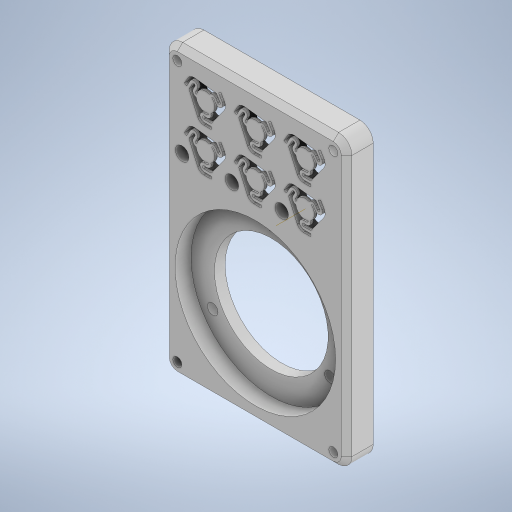
# Autodesk Inventor part: Case Front
Saved by Autodesk Inventor 2023.1 (Build 271208000, 208)
## iProperties
Created: 2022-10-09
Part Number: Case Front
Material: Generic
Document SubType Name: Modeling
Designer: Nick
Density: 1 g/cm^3
Appearance: Default
Author: Nick
Autodesk Inventor part; units mm, degrees
(part 1 of 2)
ref_plane "YZ Plane" through (0, 0, 0) normal (1, 0, 0) x (0, 1, 0)
ref_plane "XZ Plane" through (0, 0, 0) normal (0, 1, 0) x (-1, 0, 0)
ref_plane "XY Plane" through (0, 0, 0) normal (0, 0, 1) x (1, 0, 0)
sketch "Sketch1" plane through (0, 0, 0) normal (0, 0, 1) x (1, 0, 0)
  line L0 (0, 0) -> (68.58, 0)
  line L1 (68.58, 0) -> (68.58, 107.95)
  line L2 (68.58, 107.95) -> (0, 107.95)
  line L3 (0, 107.95) -> (0, 0)
  dimension "d0" = 68.58
  dimension "d1" = 107.95
  constraints: 8 end point, 2 parallel, 1 horizontal, 1 perpendicular
  measures "d0" distance of L2.end L1.end
  measures "d1" distance of L1.end L0.end
extrude "Extrusion1" add sketch "Sketch1" along normal blind 10
sketch "Sketch2" plane through (0, 0, 10) normal (0, 0, 1) x (1, 0, 0)
  circle A0 centre (34.29, 35.56) radius 30.149
  line L0 (0, 0) -> (68.58, 0) projected
  point P0 (34.29, 0)
  dimension "d4" = 60.298
  dimension "d5" = 35.56
  constraints: 1 centre point, 1 midpoint, 1 vertical alignment
  measures "d4" diameter of A0
  measures "d5" distance from line of L0 A0.centre
extrude "Extrusion2" cut sketch "Sketch2" against normal blind 16.9875
sketch "Sketch3" plane through (0, 0, 0) normal (0, 0, -1) x (-1, 0, 0)
  circle A0 centre (-34.29, 35.56) radius 30.149 projected
  circle A1 centre (-34.29, 35.56) radius 21.3606
  point P0 (0, 0)
  dimension "d8" = 42.7212
  constraints: 1 centre point, 1 coincident
  measures "d8" diameter of A1
extrude "Extrusion3" add sketch "Sketch3" against normal blind 4
sketch "Sketch4" plane through (0, 0, 10) normal (0, 0, 1) x (1, 0, 0)
  circle A0 centre (15.59, 78.7495) radius 3
  circle A1 centre (34.29, 78.7495) radius 3
  circle A2 centre (52.99, 94.9095) radius 3
  circle A3 centre (34.29, 94.9095) radius 3
  circle A4 centre (15.59, 94.9095) radius 3
  line L0 (12.59, 97.9095) -> (18.59, 97.9095) construction
  line L1 (18.59, 97.9095) -> (18.59, 91.9095) construction
  line L2 (18.59, 91.9095) -> (12.59, 91.9095) construction
  line L3 (12.59, 91.9095) -> (12.59, 97.9095) construction
  line L4 (31.29, 97.9095) -> (37.29, 97.9095) construction
  line L5 (37.29, 97.9095) -> (37.29, 91.9095) construction
  line L6 (37.29, 91.9095) -> (31.29, 91.9095) construction
  line L7 (31.29, 91.9095) -> (31.29, 97.9095) construction
  line L8 (49.99, 97.9095) -> (55.99, 97.9095) construction
  line L9 (55.99, 97.9095) -> (55.99, 91.9095) construction
  line L10 (55.99, 91.9095) -> (49.99, 91.9095) construction
  line L11 (49.99, 91.9095) -> (49.99, 97.9095) construction
  line L12 (31.29, 81.7495) -> (37.29, 81.7495) construction
  line L13 (37.29, 81.7495) -> (37.29, 75.7495) construction
  line L14 (37.29, 75.7495) -> (31.29, 75.7495) construction
  line L15 (31.29, 75.7495) -> (31.29, 81.7495) construction
  line L16 (12.59, 81.7495) -> (18.59, 81.7495) construction
  line L17 (18.59, 81.7495) -> (18.59, 75.7495) construction
  line L18 (18.59, 75.7495) -> (12.59, 75.7495) construction
  line L19 (12.59, 75.7495) -> (12.59, 81.7495) construction
  line L20 (68.58, 107.95) -> (0, 107.95) construction
  line L21 (17.8543, 65.709) -> (37.2658, 65.709) construction
  circle A5 centre (34.29, 35.56) radius 30.149 construction
  circle A6 centre (52.99, 78.7495) radius 3
  line L22 (49.99, 81.7495) -> (55.99, 81.7495) construction
  line L23 (55.99, 81.7495) -> (55.99, 75.7495) construction
  line L24 (55.99, 75.7495) -> (49.99, 75.7495) construction
  line L25 (49.99, 75.7495) -> (49.99, 81.7495) construction
  line L26 (46.7767, 79.8715) -> (48.1617, 82.2704)
  line L27 (49.2587, 80.1705) -> (49.8937, 81.2704)
  line L28 (45.9106, 80.3715) -> (47.2956, 82.7704)
  line L29 (48.3927, 80.6705) -> (49.0277, 81.7704)
  arc A7 (49.8937, 81.2704) -> (47.2956, 82.7704) centre (48.5947, 82.0204) ccw
  arc A8 (49.0277, 81.7704) -> (48.1617, 82.2704) centre (48.5947, 82.0204) ccw
  arc A9 (48.3927, 80.6705) -> (50.0046, 78.4535) centre (49.6917, 79.9205) ccw
  arc A10 (49.2587, 80.1705) -> (50.1629, 79.7532) centre (49.6917, 79.9205) ccw
  line L30 (52.99, 78.7495) -> (49.5762, 80.7205) construction
  line L31 (52.99, 81.7495) -> (52.99, 78.7495) construction
  line L32 (45.9106, 80.3715) -> (46.7767, 79.8715)
  circle A11 centre (52.99, 78.7495) radius 3.508
  line L33 (46.7767, 79.8715) -> (48.9417, 78.6215)
  line L34 (45.9106, 80.3715) -> (45.0446, 80.8715)
  line L35 (45.0446, 80.8715) -> (46.4296, 83.2704)
  arc A12 (50.7343, 80.7273) -> (46.4296, 83.2704) centre (48.5947, 82.0204) ccw
  point P0 (0, 0)
  point P1 (37.29, 78.7495)
  point P2 (18.59, 78.7495)
  point P3 (18.59, 94.9095)
  point P4 (31.29, 94.9095)
  point P5 (55.99, 94.9095)
  point P6 (34.29, 97.9095)
  point P7 (52.99, 97.9095)
  point P8 (15.59, 97.9095)
  point P9 (15.59, 81.7495)
  point P10 (34.29, 107.95)
  point P11 (55.99, 78.7495)
  point P12 (46.3436, 80.1215)
  point P13 (50.432, 77.1821)
  point P14 (49.5508, 79.4408)
  point P15 (51.0723, 81.6869)
  dimension "d11" = 10.16
  dimension "d12" = 6
  dimension "d13" = 6
  dimension "d14" = 12.7
  dimension "d15" = 12.7
  dimension "d16" = 10.0405
  dimension "d17" = 10.0405
  dimension "d34" = 6
  dimension "d35" = 6
  dimension "d36" = 1
  dimension "d37" = 60
  dimension "d38" = 1.27
  dimension "d58" = 0.508
  dimension "d129" = 1
  dimension "d131" = 1
  constraints: 70 end point, 15 parallel, 15 point on circle, 14 midpoint, 12 centre point, 11 tangent, 10 equal length, 9 perpendicular, 7 horizontal, 7 vertical alignment, 6 horizontal alignment, 5 collinear, 5 equal radius, 3 concentric, 3 point on line, 1 vertical
  measures "d11" distance between parallel lines of L12 L6
  measures "d12" distance of L12.start L12.end
  measures "d13" diameter of A1
  measures "d14" distance between parallel lines of L11 L5
  measures "d15" distance between parallel lines of L1 L7
  measures "d16" distance between parallel lines of L20 L4
  measures "d17" distance between parallel lines of L21 L14
  measures "d34" distance of L25.end L23.start
  measures "d35" diameter of A6
  measures "d36" distance between parallel lines of L27 L29
  measures "d37" angle of L31 L30
  measures "d38" distance of L29.start L29.end
  measures "d58" radial gap between concentric circles of A6 A11
  measures "d129" distance between parallel lines of L29 L26
  measures "d131" distance between parallel lines of L35 L28
extrude "Extrusion5" cut sketch "Sketch4" against normal through all contours A11 A10 L27 A7 L28 L34 L35 A12 | L33 L26 A8 L29 A9
pattern_circular "Circular Pattern2" count 3 over 360 about axis through (52.99, 78.7495, 10) along (0, 0, 1) of "Extrusion5"
sketch "Sketch6" plane through (0, 0, 10) normal (0, 0, 1) x (1, 0, 0)
  line L0 (57.0683, 83.5694) -> (58.4533, 81.1705) projected
  arc A0 (57.5873, 80.6705) -> (58.4533, 81.1705) centre (58.0203, 80.9205) ccw projected
  line L1 (57.5873, 80.6705) -> (56.9523, 81.7704) projected
  arc A1 (56.9523, 81.7704) -> (54.9033, 82.3194) centre (55.6533, 81.0204) ccw projected
  arc A2 (56.0863, 81.2704) -> (55.3083, 81.3823) centre (55.6533, 81.0204) ccw projected
  line L2 (56.0863, 81.2704) -> (56.7213, 80.1705) projected
  arc A3 (56.7213, 80.1705) -> (59.3194, 81.6705) centre (58.0203, 80.9205) ccw projected
  line L3 (59.3194, 81.6705) -> (57.9344, 84.0694) projected
  line L4 (55.125, 72.8076) -> (52.355, 72.8076) projected
  arc A4 (52.355, 73.8076) -> (52.355, 72.8076) centre (52.355, 73.3076) ccw projected
  line L5 (52.355, 73.8076) -> (53.625, 73.8076) projected
  arc A5 (53.625, 73.8076) -> (55.125, 75.3076) centre (53.625, 75.3076) ccw projected
  arc A6 (53.625, 74.8076) -> (54.1109, 75.4254) centre (53.625, 75.3076) ccw projected
  line L6 (53.625, 74.8076) -> (52.355, 74.8076) projected
  arc A7 (52.355, 74.8076) -> (52.355, 71.8076) centre (52.355, 73.3076) ccw projected
  line L7 (52.355, 71.8076) -> (55.125, 71.8076) projected
  line L8 (46.7767, 79.8715) -> (48.1617, 82.2704) projected
  arc A8 (49.0277, 81.7704) -> (48.1617, 82.2704) centre (48.5947, 82.0204) ccw projected
  line L9 (49.0277, 81.7704) -> (48.3927, 80.6705) projected
  arc A9 (48.3927, 80.6705) -> (48.9417, 78.6215) centre (49.6917, 79.9205) ccw projected
  line L10 (47.2956, 82.7704) -> (45.9106, 80.3715) projected
  arc A10 (49.2587, 80.1705) -> (49.5508, 79.4408) centre (49.6917, 79.9205) ccw projected
  line L11 (49.2587, 80.1705) -> (49.8937, 81.2704) projected
  arc A11 (49.8937, 81.2704) -> (47.2956, 82.7704) centre (48.5947, 82.0204) ccw projected
  circle A12 centre (34.29, 35.56) radius 30.149 projected
  line L12 (68.58, 0) -> (68.58, 107.95) projected
  line L13 (68.58, 107.95) -> (0, 107.95) projected
  line L14 (0, 107.95) -> (0, 0) projected
  line L15 (0, 0) -> (68.58, 0) projected
  line L16 (48.8782, 84.5043) -> (57.0683, 83.5694)
  line L17 (46.7767, 79.8715) -> (50.0621, 72.3112)
  line L18 (55.125, 72.8076) -> (60.0297, 79.4331)
  line L19 (54.9033, 82.3194) -> (57.0683, 83.5694) projected
  line L20 (57.9344, 84.0694) -> (58.8004, 84.5694) projected
  line L21 (58.8004, 84.5694) -> (60.1854, 82.1705) projected
  arc A13 (56.4927, 78.9415) -> (60.1854, 82.1705) centre (58.0203, 80.9205) ccw projected
  arc A14 (56.4927, 78.9415) -> (55.3083, 81.3823) centre (52.99, 78.7495) ccw projected
  line L22 (55.125, 75.3076) -> (55.125, 72.8076) projected
  line L23 (55.125, 71.8076) -> (55.125, 70.8076) projected
  line L24 (55.125, 70.8076) -> (52.355, 70.8076) projected
  arc A15 (51.4049, 75.62) -> (52.355, 70.8076) centre (52.355, 73.3076) ccw projected
  arc A16 (51.4049, 75.62) -> (54.1109, 75.4254) centre (52.99, 78.7495) ccw projected
  line L25 (48.9417, 78.6215) -> (46.7767, 79.8715) projected
  line L26 (45.9106, 80.3715) -> (45.0446, 80.8715) projected
  line L27 (45.0446, 80.8715) -> (46.4296, 83.2704) projected
  arc A17 (51.0723, 81.6869) -> (46.4296, 83.2704) centre (48.5947, 82.0204) ccw projected
  arc A18 (51.0723, 81.6869) -> (49.5508, 79.4408) centre (52.99, 78.7495) ccw projected
  arc A19 (51.0723, 81.6869) -> (49.5508, 79.4408) centre (52.99, 78.7495) ccw projected
  arc A20 (51.0723, 81.6869) -> (46.4296, 83.2704) centre (48.5947, 82.0204) ccw projected
  arc A21 (51.4049, 75.62) -> (52.355, 70.8076) centre (52.355, 73.3076) ccw projected
  arc A22 (48.3927, 80.6705) -> (48.9417, 78.6215) centre (49.6917, 79.9205) ccw projected
  arc A23 (48.3927, 80.6705) -> (50.0046, 78.4535) centre (49.6917, 79.9205) ccw projected
  circle A24 centre (52.99, 78.7495) radius 3.508 projected
  point P0 (49.4963, 78.4333)
  constraints: 6 end point, 3 point on circle, 3 tangent, 2 point on line
extrude "Extrusion7" cut sketch "Sketch6" against normal through all contours A24 A15 L17 L25 A23
pattern_circular "Circular Pattern3" count 3 over 360 about axis through (52.99, 78.7495, 10) along (0, 0, 1) of "Extrusion7"
pattern_linear "Rectangular Pattern2" count 3 spacing 18.7 along (-1, 0, 0) count 2 spacing 16.16 along (0, 1, 0) of "Extrusion5", "Circular Pattern2", "Extrusion7", "Circular Pattern3"
sketch "Sketch5" plane through (0, 0, 0) normal (0, 0, -1) x (-1, 0, 0)
  line L0 (-65.58, 104.95) -> (-3, 104.95)
  line L1 (-3, 104.95) -> (-3, 66.587)
  line L2 (-3, 66.587) -> (-65.58, 66.587)
  line L3 (-65.58, 66.587) -> (-65.58, 104.95)
  line L4 (-68.58, 107.95) -> (0, 107.95) projected
  line L5 (0, 107.95) -> (0, 0) projected
  line L6 (-68.58, 0) -> (-68.58, 107.95) projected
  line L7 (-14.955, 70.8076) -> (-17.725, 70.8076) projected
  point P0 (-21.4004, 100.7294)
  point P1 (-21.4004, 100.7294)
  dimension "d52" = 3
  dimension "d53" = 3
  dimension "d54" = 3
  dimension "d74" = 4.2206
  dimension "d136" = 4.2206
  constraints: 8 end point, 2 parallel, 1 coincident, 1 horizontal, 1 perpendicular
  measures "d52" distance between parallel lines of L4 L0
  measures "d53" distance between parallel lines of L5 L1
  measures "d54" distance between parallel lines of L6 L3
  measures "d74" distance from line of L0 point (-21.4, 100.729)
  measures "d136" distance between parallel lines of L2 L7
extrude "Extrusion6" cut sketch "Sketch5" against normal blind 9
sketch "Sketch7" plane through (0, 0, 10) normal (0, 0, 1) x (1, 0, 0)
  line L0 (13.1513, 70.2434) -> (18.0287, 70.2434) construction
  line L1 (18.0287, 70.2434) -> (18.0287, 66.7015) construction
  line L2 (18.0287, 66.7015) -> (13.1513, 66.7015) construction
  line L3 (13.1513, 66.7015) -> (13.1513, 70.2434) construction
  line L4 (31.7583, 70.2434) -> (36.8217, 70.2434) construction
  line L5 (36.8217, 70.2434) -> (36.8217, 66.7015) construction
  line L6 (36.8217, 66.7015) -> (31.7583, 66.7015) construction
  line L7 (31.7583, 66.7015) -> (31.7583, 70.2434) construction
  line L8 (53.7679, 70.2434) -> (52.2121, 70.2434) construction
  line L9 (52.2121, 70.2434) -> (52.2121, 66.7015) construction
  line L10 (52.2121, 66.7015) -> (53.7679, 66.7015) construction
  line L11 (53.7679, 66.7015) -> (53.7679, 70.2434) construction
  line L12 (12.8075, 104.5617) -> (18.3725, 104.5617) construction
  line L13 (18.3725, 104.5617) -> (18.3725, 101.405) construction
  line L14 (18.3725, 101.405) -> (12.8075, 101.405) construction
  line L15 (12.8075, 101.405) -> (12.8075, 104.5617) construction
  line L16 (31.3295, 104.5617) -> (37.2505, 104.5617) construction
  line L17 (37.2505, 104.5617) -> (37.2505, 101.405) construction
  line L18 (37.2505, 101.405) -> (31.3295, 101.405) construction
  line L19 (31.3295, 101.405) -> (31.3295, 104.5617) construction
  line L20 (49.6833, 104.5617) -> (56.2967, 104.5617) construction
  line L21 (56.2967, 104.5617) -> (56.2967, 101.405) construction
  line L22 (56.2967, 101.405) -> (49.6833, 101.405) construction
  line L23 (49.6833, 101.405) -> (49.6833, 104.5617) construction
  line L24 (68.58, 0) -> (68.58, 107.95) projected
  line L25 (68.58, 107.95) -> (0, 107.95) projected
  line L26 (0, 107.95) -> (0, 0) projected
  line L27 (0, 0) -> (68.58, 0) projected
  circle A0 centre (34.29, 35.56) radius 30.149 projected
  line L28 (57.0683, 83.5694) -> (58.4533, 81.1705) projected
  arc A1 (57.5873, 80.6705) -> (58.4533, 81.1705) centre (58.0203, 80.9205) ccw projected
  line L29 (57.5873, 80.6705) -> (56.9523, 81.7704) projected
  arc A2 (56.9523, 81.7704) -> (54.463, 81.9332) centre (55.6533, 81.0204) ccw projected
  arc A3 (49.2587, 80.1705) -> (49.5508, 79.4408) centre (49.6917, 79.9205) ccw projected
  line L30 (49.2587, 80.1705) -> (49.8937, 81.2704) projected
  arc A4 (49.8937, 81.2704) -> (47.2956, 82.7704) centre (48.5947, 82.0204) ccw projected
  line L31 (47.2956, 82.7704) -> (45.9106, 80.3715) projected
  line L32 (55.125, 72.8076) -> (52.355, 72.8076) projected
  arc A5 (52.355, 73.8076) -> (52.355, 72.8076) centre (52.355, 73.3076) ccw projected
  line L33 (52.355, 73.8076) -> (53.625, 73.8076) projected
  arc A6 (53.625, 73.8076) -> (55.0107, 75.8819) centre (53.625, 75.3076) ccw projected
  arc A7 (56.0863, 81.2704) -> (55.3083, 81.3823) centre (55.6533, 81.0204) ccw projected
  line L34 (56.0863, 81.2704) -> (56.7213, 80.1705) projected
  arc A8 (56.7213, 80.1705) -> (59.3194, 81.6705) centre (58.0203, 80.9205) ccw projected
  line L35 (59.3194, 81.6705) -> (57.9344, 84.0694) projected
  line L36 (46.7767, 79.8715) -> (48.1617, 82.2704) projected
  arc A9 (49.0277, 81.7704) -> (48.1617, 82.2704) centre (48.5947, 82.0204) ccw projected
  line L37 (49.0277, 81.7704) -> (48.3927, 80.6705) projected
  arc A10 (48.3927, 80.6705) -> (49.4963, 78.4333) centre (49.6917, 79.9205) ccw projected
  arc A11 (53.625, 74.8076) -> (54.1109, 75.4254) centre (53.625, 75.3076) ccw projected
  line L38 (53.625, 74.8076) -> (52.355, 74.8076) projected
  arc A12 (52.355, 74.8076) -> (52.355, 71.8076) centre (52.355, 73.3076) ccw projected
  line L39 (52.355, 71.8076) -> (55.125, 71.8076) projected
  arc A13 (34.925, 74.8076) -> (35.4109, 75.4254) centre (34.925, 75.3076) ccw projected
  line L40 (34.925, 74.8076) -> (33.655, 74.8076) projected
  arc A14 (33.655, 74.8076) -> (33.655, 71.8076) centre (33.655, 73.3076) ccw projected
  line L41 (33.655, 71.8076) -> (36.425, 71.8076) projected
  line L42 (28.0767, 79.8715) -> (29.4617, 82.2704) projected
  arc A15 (30.3277, 81.7704) -> (29.4617, 82.2704) centre (29.8947, 82.0204) ccw projected
  line L43 (30.3277, 81.7704) -> (29.6927, 80.6705) projected
  arc A16 (29.6927, 80.6705) -> (30.7963, 78.4333) centre (30.9917, 79.9205) ccw projected
  arc A17 (37.3863, 81.2704) -> (36.6083, 81.3823) centre (36.9533, 81.0204) ccw projected
  line L44 (37.3863, 81.2704) -> (38.0213, 80.1705) projected
  arc A18 (38.0213, 80.1705) -> (40.6194, 81.6705) centre (39.3203, 80.9205) ccw projected
  line L45 (40.6194, 81.6705) -> (39.2344, 84.0694) projected
  line L46 (36.425, 72.8076) -> (33.655, 72.8076) projected
  arc A19 (33.655, 73.8076) -> (33.655, 72.8076) centre (33.655, 73.3076) ccw projected
  line L47 (33.655, 73.8076) -> (34.925, 73.8076) projected
  arc A20 (34.925, 73.8076) -> (36.3107, 75.8819) centre (34.925, 75.3076) ccw projected
  line L48 (38.3683, 83.5694) -> (39.7533, 81.1705) projected
  arc A21 (38.8873, 80.6705) -> (39.7533, 81.1705) centre (39.3203, 80.9205) ccw projected
  line L49 (38.8873, 80.6705) -> (38.2523, 81.7704) projected
  arc A22 (38.2523, 81.7704) -> (35.763, 81.9332) centre (36.9533, 81.0204) ccw projected
  arc A23 (30.5587, 80.1705) -> (30.8508, 79.4408) centre (30.9917, 79.9205) ccw projected
  line L50 (30.5587, 80.1705) -> (31.1937, 81.2704) projected
  arc A24 (31.1937, 81.2704) -> (28.5956, 82.7704) centre (29.8947, 82.0204) ccw projected
  line L51 (28.5956, 82.7704) -> (27.2106, 80.3715) projected
  arc A25 (16.225, 74.8076) -> (16.7109, 75.4254) centre (16.225, 75.3076) ccw projected
  line L52 (16.225, 74.8076) -> (14.955, 74.8076) projected
  arc A26 (14.955, 74.8076) -> (14.955, 71.8076) centre (14.955, 73.3076) ccw projected
  line L53 (14.955, 71.8076) -> (17.725, 71.8076) projected
  line L54 (9.3767, 79.8715) -> (10.7617, 82.2704) projected
  arc A27 (11.6277, 81.7704) -> (10.7617, 82.2704) centre (11.1947, 82.0204) ccw projected
  line L55 (11.6277, 81.7704) -> (10.9927, 80.6705) projected
  arc A28 (10.9927, 80.6705) -> (12.0963, 78.4333) centre (12.2917, 79.9205) ccw projected
  arc A29 (18.6863, 81.2704) -> (17.9083, 81.3823) centre (18.2533, 81.0204) ccw projected
  line L56 (18.6863, 81.2704) -> (19.3213, 80.1705) projected
  arc A30 (19.3213, 80.1705) -> (21.9194, 81.6705) centre (20.6203, 80.9205) ccw projected
  line L57 (21.9194, 81.6705) -> (20.5344, 84.0694) projected
  line L58 (17.725, 72.8076) -> (14.955, 72.8076) projected
  arc A31 (14.955, 73.8076) -> (14.955, 72.8076) centre (14.955, 73.3076) ccw projected
  line L59 (14.955, 73.8076) -> (16.225, 73.8076) projected
  arc A32 (16.225, 73.8076) -> (17.6107, 75.8819) centre (16.225, 75.3076) ccw projected
  line L60 (19.6683, 83.5694) -> (21.0533, 81.1705) projected
  arc A33 (20.1873, 80.6705) -> (21.0533, 81.1705) centre (20.6203, 80.9205) ccw projected
  line L61 (20.1873, 80.6705) -> (19.5523, 81.7704) projected
  arc A34 (19.5523, 81.7704) -> (17.063, 81.9332) centre (18.2533, 81.0204) ccw projected
  arc A35 (11.8587, 80.1705) -> (12.1508, 79.4408) centre (12.2917, 79.9205) ccw projected
  line L62 (11.8587, 80.1705) -> (12.4937, 81.2704) projected
  arc A36 (12.4937, 81.2704) -> (9.8956, 82.7704) centre (11.1947, 82.0204) ccw projected
  line L63 (9.8956, 82.7704) -> (8.5106, 80.3715) projected
  arc A37 (53.625, 90.9676) -> (54.1109, 91.5854) centre (53.625, 91.4676) ccw projected
  line L64 (53.625, 90.9676) -> (52.355, 90.9676) projected
  arc A38 (52.355, 90.9676) -> (52.355, 87.9676) centre (52.355, 89.4676) ccw projected
  line L65 (52.355, 87.9676) -> (55.125, 87.9676) projected
  line L66 (46.7767, 96.0315) -> (48.1617, 98.4304) projected
  arc A39 (49.0277, 97.9304) -> (48.1617, 98.4304) centre (48.5947, 98.1804) ccw projected
  line L67 (49.0277, 97.9304) -> (48.3927, 96.8305) projected
  arc A40 (48.3927, 96.8305) -> (49.4963, 94.5933) centre (49.6917, 96.0805) ccw projected
  arc A41 (56.0863, 97.4304) -> (55.3083, 97.5423) centre (55.6533, 97.1804) ccw projected
  line L68 (56.0863, 97.4304) -> (56.7213, 96.3305) projected
  arc A42 (56.7213, 96.3305) -> (59.3194, 97.8305) centre (58.0203, 97.0805) ccw projected
  line L69 (59.3194, 97.8305) -> (57.9344, 100.2294) projected
  line L70 (55.125, 88.9676) -> (52.355, 88.9676) projected
  arc A43 (52.355, 89.9676) -> (52.355, 88.9676) centre (52.355, 89.4676) ccw projected
  line L71 (52.355, 89.9676) -> (53.625, 89.9676) projected
  arc A44 (53.625, 89.9676) -> (55.0107, 92.0419) centre (53.625, 91.4676) ccw projected
  line L72 (57.0683, 99.7294) -> (58.4533, 97.3305) projected
  arc A45 (57.5873, 96.8305) -> (58.4533, 97.3305) centre (58.0203, 97.0805) ccw projected
  line L73 (57.5873, 96.8305) -> (56.9523, 97.9304) projected
  arc A46 (56.9523, 97.9304) -> (54.463, 98.0932) centre (55.6533, 97.1804) ccw projected
  arc A47 (49.2587, 96.3305) -> (49.5508, 95.6008) centre (49.6917, 96.0805) ccw projected
  line L74 (49.2587, 96.3305) -> (49.8937, 97.4304) projected
  arc A48 (49.8937, 97.4304) -> (47.2956, 98.9304) centre (48.5947, 98.1804) ccw projected
  line L75 (47.2956, 98.9304) -> (45.9106, 96.5315) projected
  arc A49 (34.925, 90.9676) -> (35.4109, 91.5854) centre (34.925, 91.4676) ccw projected
  line L76 (34.925, 90.9676) -> (33.655, 90.9676) projected
  arc A50 (33.655, 90.9676) -> (33.655, 87.9676) centre (33.655, 89.4676) ccw projected
  line L77 (33.655, 87.9676) -> (36.425, 87.9676) projected
  line L78 (28.0767, 96.0315) -> (29.4617, 98.4304) projected
  arc A51 (30.3277, 97.9304) -> (29.4617, 98.4304) centre (29.8947, 98.1804) ccw projected
  line L79 (30.3277, 97.9304) -> (29.6927, 96.8305) projected
  arc A52 (29.6927, 96.8305) -> (30.7963, 94.5933) centre (30.9917, 96.0805) ccw projected
  arc A53 (37.3863, 97.4304) -> (36.6083, 97.5423) centre (36.9533, 97.1804) ccw projected
  line L80 (37.3863, 97.4304) -> (38.0213, 96.3305) projected
  arc A54 (38.0213, 96.3305) -> (40.6194, 97.8305) centre (39.3203, 97.0805) ccw projected
  line L81 (40.6194, 97.8305) -> (39.2344, 100.2294) projected
  line L82 (36.425, 88.9676) -> (33.655, 88.9676) projected
  arc A55 (33.655, 89.9676) -> (33.655, 88.9676) centre (33.655, 89.4676) ccw projected
  line L83 (33.655, 89.9676) -> (34.925, 89.9676) projected
  arc A56 (34.925, 89.9676) -> (36.3107, 92.0419) centre (34.925, 91.4676) ccw projected
  line L84 (38.3683, 99.7294) -> (39.7533, 97.3305) projected
  arc A57 (38.8873, 96.8305) -> (39.7533, 97.3305) centre (39.3203, 97.0805) ccw projected
  line L85 (38.8873, 96.8305) -> (38.2523, 97.9304) projected
  arc A58 (38.2523, 97.9304) -> (35.763, 98.0932) centre (36.9533, 97.1804) ccw projected
  arc A59 (30.5587, 96.3305) -> (30.8508, 95.6008) centre (30.9917, 96.0805) ccw projected
  line L86 (30.5587, 96.3305) -> (31.1937, 97.4304) projected
  arc A60 (31.1937, 97.4304) -> (28.5956, 98.9304) centre (29.8947, 98.1804) ccw projected
  line L87 (28.5956, 98.9304) -> (27.2106, 96.5315) projected
  arc A61 (16.225, 90.9676) -> (16.7109, 91.5854) centre (16.225, 91.4676) ccw projected
  line L88 (16.225, 90.9676) -> (14.955, 90.9676) projected
  arc A62 (14.955, 90.9676) -> (14.955, 87.9676) centre (14.955, 89.4676) ccw projected
  line L89 (14.955, 87.9676) -> (17.725, 87.9676) projected
  line L90 (9.3767, 96.0315) -> (10.7617, 98.4304) projected
  arc A63 (11.6277, 97.9304) -> (10.7617, 98.4304) centre (11.1947, 98.1804) ccw projected
  line L91 (11.6277, 97.9304) -> (10.9927, 96.8305) projected
  arc A64 (10.9927, 96.8305) -> (12.0963, 94.5933) centre (12.2917, 96.0805) ccw projected
  arc A65 (18.6863, 97.4304) -> (17.9083, 97.5423) centre (18.2533, 97.1804) ccw projected
  line L92 (18.6863, 97.4304) -> (19.3213, 96.3305) projected
  arc A66 (19.3213, 96.3305) -> (21.9194, 97.8305) centre (20.6203, 97.0805) ccw projected
  line L93 (21.9194, 97.8305) -> (20.5344, 100.2294) projected
  line L94 (17.725, 88.9676) -> (14.955, 88.9676) projected
  arc A67 (14.955, 89.9676) -> (14.955, 88.9676) centre (14.955, 89.4676) ccw projected
  line L95 (14.955, 89.9676) -> (16.225, 89.9676) projected
  arc A68 (16.225, 89.9676) -> (17.6107, 92.0419) centre (16.225, 91.4676) ccw projected
  line L96 (19.6683, 99.7294) -> (21.0533, 97.3305) projected
  arc A69 (20.1873, 96.8305) -> (21.0533, 97.3305) centre (20.6203, 97.0805) ccw projected
  line L97 (20.1873, 96.8305) -> (19.5523, 97.9304) projected
  arc A70 (19.5523, 97.9304) -> (17.063, 98.0932) centre (18.2533, 97.1804) ccw projected
  arc A71 (11.8587, 96.3305) -> (12.1508, 95.6008) centre (12.2917, 96.0805) ccw projected
  line L98 (11.8587, 96.3305) -> (12.4937, 97.4304) projected
  arc A72 (12.4937, 97.4304) -> (9.8956, 98.9304) centre (11.1947, 98.1804) ccw projected
  line L99 (9.8956, 98.9304) -> (8.5106, 96.5315) projected
  circle A73 centre (6.7912, 73.6695) radius 2.55
  circle A74 centre (25.4912, 73.6695) radius 2.55
  circle A75 centre (44.1912, 73.6695) radius 2.55
  line L100 (15.59, 78.7495) -> (52.99, 78.7495) construction
  line L101 (15.59, 78.7495) -> (6.7912, 73.6695) construction
  line L102 (52.99, 78.7495) -> (44.1912, 73.6695) construction
  line L103 (55.125, 71.8076) -> (55.125, 70.8076) projected
  line L104 (55.125, 70.8076) -> (52.355, 70.8076) projected
  arc A76 (50.0621, 72.3112) -> (52.355, 70.8076) centre (52.355, 73.3076) ccw projected
  line L105 (45.9106, 80.3715) -> (45.0446, 80.8715) projected
  line L106 (45.0446, 80.8715) -> (46.4296, 83.2704) projected
  arc A77 (48.8782, 84.5043) -> (46.4296, 83.2704) centre (48.5947, 82.0204) ccw projected
  line L107 (57.9344, 84.0694) -> (58.8004, 84.5694) projected
  line L108 (58.8004, 84.5694) -> (60.1854, 82.1705) projected
  arc A78 (60.0297, 79.4331) -> (60.1854, 82.1705) centre (58.0203, 80.9205) ccw projected
  arc A79 (35.763, 81.9332) -> (30.8508, 79.4408) centre (34.29, 78.7495) ccw projected
  line L109 (36.425, 71.8076) -> (36.425, 70.8076) projected
  line L110 (36.425, 70.8076) -> (33.655, 70.8076) projected
  arc A80 (31.3621, 72.3112) -> (33.655, 70.8076) centre (33.655, 73.3076) ccw projected
  line L111 (27.2106, 80.3715) -> (26.3446, 80.8715) projected
  line L112 (26.3446, 80.8715) -> (27.7296, 83.2704) projected
  arc A81 (30.1782, 84.5043) -> (27.7296, 83.2704) centre (29.8947, 82.0204) ccw projected
  line L113 (39.2344, 84.0694) -> (40.1004, 84.5694) projected
  line L114 (40.1004, 84.5694) -> (41.4854, 82.1705) projected
  arc A82 (41.3297, 79.4331) -> (41.4854, 82.1705) centre (39.3203, 80.9205) ccw projected
  arc A83 (17.063, 81.9332) -> (12.1508, 79.4408) centre (15.59, 78.7495) ccw projected
  line L115 (17.725, 71.8076) -> (17.725, 70.8076) projected
  line L116 (17.725, 70.8076) -> (14.955, 70.8076) projected
  arc A84 (12.6621, 72.3112) -> (14.955, 70.8076) centre (14.955, 73.3076) ccw projected
  line L117 (8.5106, 80.3715) -> (7.6446, 80.8715) projected
  line L118 (7.6446, 80.8715) -> (9.0296, 83.2704) projected
  arc A85 (11.4782, 84.5043) -> (9.0296, 83.2704) centre (11.1947, 82.0204) ccw projected
  line L119 (20.5344, 84.0694) -> (21.4004, 84.5694) projected
  line L120 (21.4004, 84.5694) -> (22.7854, 82.1705) projected
  arc A86 (22.6297, 79.4331) -> (22.7854, 82.1705) centre (20.6203, 80.9205) ccw projected
  arc A87 (54.463, 98.0932) -> (49.5508, 95.6008) centre (52.99, 94.9095) ccw projected
  line L121 (55.125, 87.9676) -> (55.125, 86.9676) projected
  line L122 (55.125, 86.9676) -> (52.355, 86.9676) projected
  arc A88 (50.0621, 88.4712) -> (52.355, 86.9676) centre (52.355, 89.4676) ccw projected
  line L123 (45.9106, 96.5315) -> (45.0446, 97.0315) projected
  line L124 (45.0446, 97.0315) -> (46.4296, 99.4304) projected
  arc A89 (48.8782, 100.6643) -> (46.4296, 99.4304) centre (48.5947, 98.1804) ccw projected
  line L125 (57.9344, 100.2294) -> (58.8004, 100.7294) projected
  line L126 (58.8004, 100.7294) -> (60.1854, 98.3305) projected
  arc A90 (60.0297, 95.5931) -> (60.1854, 98.3305) centre (58.0203, 97.0805) ccw projected
  arc A91 (35.763, 98.0932) -> (30.8508, 95.6008) centre (34.29, 94.9095) ccw projected
  line L127 (36.425, 87.9676) -> (36.425, 86.9676) projected
  line L128 (36.425, 86.9676) -> (33.655, 86.9676) projected
  arc A92 (31.3621, 88.4712) -> (33.655, 86.9676) centre (33.655, 89.4676) ccw projected
  line L129 (27.2106, 96.5315) -> (26.3446, 97.0315) projected
  line L130 (26.3446, 97.0315) -> (27.7296, 99.4304) projected
  arc A93 (30.1782, 100.6643) -> (27.7296, 99.4304) centre (29.8947, 98.1804) ccw projected
  line L131 (39.2344, 100.2294) -> (40.1004, 100.7294) projected
  line L132 (40.1004, 100.7294) -> (41.4854, 98.3305) projected
  arc A94 (41.3297, 95.5931) -> (41.4854, 98.3305) centre (39.3203, 97.0805) ccw projected
  arc A95 (17.063, 98.0932) -> (12.1508, 95.6008) centre (15.59, 94.9095) ccw projected
  line L133 (17.725, 87.9676) -> (17.725, 86.9676) projected
  line L134 (17.725, 86.9676) -> (14.955, 86.9676) projected
  arc A96 (12.6621, 88.4712) -> (14.955, 86.9676) centre (14.955, 89.4676) ccw projected
  line L135 (8.5106, 96.5315) -> (7.6446, 97.0315) projected
  line L136 (7.6446, 97.0315) -> (9.0296, 99.4304) projected
  arc A97 (11.4782, 100.6643) -> (9.0296, 99.4304) centre (11.1947, 98.1804) ccw projected
  line L137 (20.5344, 100.2294) -> (21.4004, 100.7294) projected
  line L138 (21.4004, 100.7294) -> (22.7854, 98.3305) projected
  arc A98 (22.6297, 95.5931) -> (22.7854, 98.3305) centre (20.6203, 97.0805) ccw projected
  arc A99 (12.0963, 94.5933) -> (16.7109, 91.5854) centre (15.59, 94.9095) ccw projected
  line L139 (12.6621, 88.4712) -> (9.3767, 96.0315) projected
  arc A100 (30.7963, 94.5933) -> (35.4109, 91.5854) centre (34.29, 94.9095) ccw projected
  line L140 (31.3621, 88.4712) -> (28.0767, 96.0315) projected
  arc A101 (49.4963, 94.5933) -> (54.1109, 91.5854) centre (52.99, 94.9095) ccw projected
  line L141 (50.0621, 88.4712) -> (46.7767, 96.0315) projected
  arc A102 (12.0963, 78.4333) -> (16.7109, 75.4254) centre (15.59, 78.7495) ccw projected
  line L142 (12.6621, 72.3112) -> (9.3767, 79.8715) projected
  arc A103 (30.7963, 78.4333) -> (35.4109, 75.4254) centre (34.29, 78.7495) ccw projected
  line L143 (31.3621, 72.3112) -> (28.0767, 79.8715) projected
  arc A104 (17.6107, 92.0419) -> (17.9083, 97.5423) centre (15.59, 94.9095) ccw projected
  arc A105 (36.3107, 92.0419) -> (36.6083, 97.5423) centre (34.29, 94.9095) ccw projected
  arc A106 (55.0107, 92.0419) -> (55.3083, 97.5423) centre (52.99, 94.9095) ccw projected
  arc A107 (17.6107, 75.8819) -> (17.9083, 81.3823) centre (15.59, 78.7495) ccw projected
  arc A108 (36.3107, 75.8819) -> (36.6083, 81.3823) centre (34.29, 78.7495) ccw projected
  arc A109 (54.463, 81.9332) -> (49.5508, 79.4408) centre (52.99, 78.7495) ccw projected
  line L144 (48.8782, 84.5043) -> (57.0683, 83.5694) projected
  arc A110 (55.0107, 75.8819) -> (55.3083, 81.3823) centre (52.99, 78.7495) ccw projected
  line L145 (60.0297, 79.4331) -> (55.125, 72.8076) projected
  line L146 (50.0621, 72.3112) -> (46.7767, 79.8715) projected
  arc A111 (49.4963, 78.4333) -> (54.1109, 75.4254) centre (52.99, 78.7495) ccw projected
  line L147 (25.4912, 73.6695) -> (34.29, 78.7495) construction
  line L148 (11.4782, 100.6643) -> (19.6683, 99.7294) projected
  line L149 (22.6297, 95.5931) -> (17.725, 88.9676) projected
  line L150 (30.1782, 100.6643) -> (38.3683, 99.7294) projected
  line L151 (41.3297, 95.5931) -> (36.425, 88.9676) projected
  line L152 (48.8782, 100.6643) -> (57.0683, 99.7294) projected
  line L153 (60.0297, 95.5931) -> (55.125, 88.9676) projected
  line L154 (11.4782, 84.5043) -> (19.6683, 83.5694) projected
  line L155 (22.6297, 79.4331) -> (17.725, 72.8076) projected
  line L156 (30.1782, 84.5043) -> (38.3683, 83.5694) projected
  line L157 (41.3297, 79.4331) -> (36.425, 72.8076) projected
  point P0 (52.99, 101.405)
  point P1 (34.29, 101.405)
  point P2 (15.59, 101.405)
  point P3 (34.29, 70.2434)
  point P4 (52.99, 70.2434)
  point P5 (15.59, 70.2434)
  dimension "d0" = 68.58
  dimension "d1" = 107.95
  dimension "d63" = 5.1
  dimension "d64" = 30
  dimension "d66" = 30
  dimension "d137" = 10.16
  constraints: 8 collinear, 8 end point, 8 vertical alignment, 7 midpoint, 3 centre point, 3 parallel, 2 coincident, 2 equal radius, 1 horizontal, 1 point on line, 12 other
  measures "d63" diameter of A73
  measures "d64" angle of L100 L102
  measures "d66" angle of L100 L101
  measures "d137" distance of L147.start L147.end
extrude "Extrusion8" cut sketch "Sketch7" against normal through all contours A73 | A74 | A75
sketch "Sketch8" plane through (0, 0, 9) normal (0, 0, -1) x (-1, 0, 0)
  circle A0 centre (-6.7912, 73.6695) radius 2.55 projected
  circle A1 centre (-44.1912, 73.6695) radius 2.55 projected
  circle A2 centre (-25.4912, 73.6695) radius 2.55 projected
  line L0 (-14.955, 87.9676) -> (-17.725, 87.9676) projected
  arc A3 (-14.955, 87.9676) -> (-14.955, 90.9676) centre (-14.955, 89.4676) ccw projected
  line L1 (-16.225, 90.9676) -> (-14.955, 90.9676) projected
  arc A4 (-16.7109, 91.5854) -> (-16.225, 90.9676) centre (-16.225, 91.4676) ccw projected
  arc A5 (-12.0963, 94.5933) -> (-10.9927, 96.8305) centre (-12.2917, 96.0805) ccw projected
  line L2 (-11.6277, 97.9304) -> (-10.9927, 96.8305) projected
  arc A6 (-10.7617, 98.4304) -> (-11.6277, 97.9304) centre (-11.1947, 98.1804) ccw projected
  line L3 (-9.3767, 96.0315) -> (-10.7617, 98.4304) projected
  line L4 (-21.9194, 97.8305) -> (-20.5344, 100.2294) projected
  arc A7 (-21.9194, 97.8305) -> (-19.3213, 96.3305) centre (-20.6203, 97.0805) ccw projected
  line L5 (-18.6863, 97.4304) -> (-19.3213, 96.3305) projected
  arc A8 (-17.9083, 97.5423) -> (-18.6863, 97.4304) centre (-18.2533, 97.1804) ccw projected
  arc A9 (-17.6107, 92.0419) -> (-16.225, 89.9676) centre (-16.225, 91.4676) ccw projected
  line L6 (-14.955, 89.9676) -> (-16.225, 89.9676) projected
  arc A10 (-14.955, 88.9676) -> (-14.955, 89.9676) centre (-14.955, 89.4676) ccw projected
  line L7 (-17.725, 88.9676) -> (-14.955, 88.9676) projected
  line L8 (-9.8956, 98.9304) -> (-8.5106, 96.5315) projected
  arc A11 (-9.8956, 98.9304) -> (-12.4937, 97.4304) centre (-11.1947, 98.1804) ccw projected
  line L9 (-11.8587, 96.3305) -> (-12.4937, 97.4304) projected
  arc A12 (-12.1508, 95.6008) -> (-11.8587, 96.3305) centre (-12.2917, 96.0805) ccw projected
  arc A13 (-17.063, 98.0932) -> (-19.5523, 97.9304) centre (-18.2533, 97.1804) ccw projected
  line L10 (-20.1873, 96.8305) -> (-19.5523, 97.9304) projected
  arc A14 (-21.0533, 97.3305) -> (-20.1873, 96.8305) centre (-20.6203, 97.0805) ccw projected
  line L11 (-19.6683, 99.7294) -> (-21.0533, 97.3305) projected
  line L12 (-33.655, 87.9676) -> (-36.425, 87.9676) projected
  arc A15 (-33.655, 87.9676) -> (-33.655, 90.9676) centre (-33.655, 89.4676) ccw projected
  line L13 (-34.925, 90.9676) -> (-33.655, 90.9676) projected
  arc A16 (-35.4109, 91.5854) -> (-34.925, 90.9676) centre (-34.925, 91.4676) ccw projected
  arc A17 (-30.7963, 94.5933) -> (-29.6927, 96.8305) centre (-30.9917, 96.0805) ccw projected
  line L14 (-30.3277, 97.9304) -> (-29.6927, 96.8305) projected
  arc A18 (-29.4617, 98.4304) -> (-30.3277, 97.9304) centre (-29.8947, 98.1804) ccw projected
  line L15 (-28.0767, 96.0315) -> (-29.4617, 98.4304) projected
  line L16 (-40.6194, 97.8305) -> (-39.2344, 100.2294) projected
  arc A19 (-40.6194, 97.8305) -> (-38.0213, 96.3305) centre (-39.3203, 97.0805) ccw projected
  line L17 (-37.3863, 97.4304) -> (-38.0213, 96.3305) projected
  arc A20 (-36.6083, 97.5423) -> (-37.3863, 97.4304) centre (-36.9533, 97.1804) ccw projected
  arc A21 (-36.3107, 92.0419) -> (-34.925, 89.9676) centre (-34.925, 91.4676) ccw projected
  line L18 (-33.655, 89.9676) -> (-34.925, 89.9676) projected
  arc A22 (-33.655, 88.9676) -> (-33.655, 89.9676) centre (-33.655, 89.4676) ccw projected
  line L19 (-36.425, 88.9676) -> (-33.655, 88.9676) projected
  line L20 (-28.5956, 98.9304) -> (-27.2106, 96.5315) projected
  arc A23 (-28.5956, 98.9304) -> (-31.1937, 97.4304) centre (-29.8947, 98.1804) ccw projected
  line L21 (-30.5587, 96.3305) -> (-31.1937, 97.4304) projected
  arc A24 (-30.8508, 95.6008) -> (-30.5587, 96.3305) centre (-30.9917, 96.0805) ccw projected
  arc A25 (-35.763, 98.0932) -> (-38.2523, 97.9304) centre (-36.9533, 97.1804) ccw projected
  line L22 (-38.8873, 96.8305) -> (-38.2523, 97.9304) projected
  arc A26 (-39.7533, 97.3305) -> (-38.8873, 96.8305) centre (-39.3203, 97.0805) ccw projected
  line L23 (-38.3683, 99.7294) -> (-39.7533, 97.3305) projected
  line L24 (-52.355, 87.9676) -> (-55.125, 87.9676) projected
  arc A27 (-52.355, 87.9676) -> (-52.355, 90.9676) centre (-52.355, 89.4676) ccw projected
  line L25 (-53.625, 90.9676) -> (-52.355, 90.9676) projected
  arc A28 (-54.1109, 91.5854) -> (-53.625, 90.9676) centre (-53.625, 91.4676) ccw projected
  arc A29 (-49.4963, 94.5933) -> (-48.3927, 96.8305) centre (-49.6917, 96.0805) ccw projected
  line L26 (-49.0277, 97.9304) -> (-48.3927, 96.8305) projected
  arc A30 (-48.1617, 98.4304) -> (-49.0277, 97.9304) centre (-48.5947, 98.1804) ccw projected
  line L27 (-46.7767, 96.0315) -> (-48.1617, 98.4304) projected
  line L28 (-59.3194, 97.8305) -> (-57.9344, 100.2294) projected
  arc A31 (-59.3194, 97.8305) -> (-56.7213, 96.3305) centre (-58.0203, 97.0805) ccw projected
  line L29 (-56.0863, 97.4304) -> (-56.7213, 96.3305) projected
  arc A32 (-55.3083, 97.5423) -> (-56.0863, 97.4304) centre (-55.6533, 97.1804) ccw projected
  arc A33 (-55.0107, 92.0419) -> (-53.625, 89.9676) centre (-53.625, 91.4676) ccw projected
  line L30 (-52.355, 89.9676) -> (-53.625, 89.9676) projected
  arc A34 (-52.355, 88.9676) -> (-52.355, 89.9676) centre (-52.355, 89.4676) ccw projected
  line L31 (-55.125, 88.9676) -> (-52.355, 88.9676) projected
  line L32 (-47.2956, 98.9304) -> (-45.9106, 96.5315) projected
  arc A35 (-47.2956, 98.9304) -> (-49.8937, 97.4304) centre (-48.5947, 98.1804) ccw projected
  line L33 (-49.2587, 96.3305) -> (-49.8937, 97.4304) projected
  arc A36 (-49.5508, 95.6008) -> (-49.2587, 96.3305) centre (-49.6917, 96.0805) ccw projected
  arc A37 (-54.463, 98.0932) -> (-56.9523, 97.9304) centre (-55.6533, 97.1804) ccw projected
  line L34 (-57.5873, 96.8305) -> (-56.9523, 97.9304) projected
  arc A38 (-58.4533, 97.3305) -> (-57.5873, 96.8305) centre (-58.0203, 97.0805) ccw projected
  line L35 (-57.0683, 99.7294) -> (-58.4533, 97.3305) projected
  line L36 (-14.955, 71.8076) -> (-17.725, 71.8076) projected
  arc A39 (-14.955, 71.8076) -> (-14.955, 74.8076) centre (-14.955, 73.3076) ccw projected
  line L37 (-16.225, 74.8076) -> (-14.955, 74.8076) projected
  arc A40 (-16.7109, 75.4254) -> (-16.225, 74.8076) centre (-16.225, 75.3076) ccw projected
  arc A41 (-12.0963, 78.4333) -> (-10.9927, 80.6705) centre (-12.2917, 79.9205) ccw projected
  line L38 (-11.6277, 81.7704) -> (-10.9927, 80.6705) projected
  arc A42 (-10.7617, 82.2704) -> (-11.6277, 81.7704) centre (-11.1947, 82.0204) ccw projected
  line L39 (-9.3767, 79.8715) -> (-10.7617, 82.2704) projected
  line L40 (-21.9194, 81.6705) -> (-20.5344, 84.0694) projected
  arc A43 (-21.9194, 81.6705) -> (-19.3213, 80.1705) centre (-20.6203, 80.9205) ccw projected
  line L41 (-18.6863, 81.2704) -> (-19.3213, 80.1705) projected
  arc A44 (-17.9083, 81.3823) -> (-18.6863, 81.2704) centre (-18.2533, 81.0204) ccw projected
  arc A45 (-17.6107, 75.8819) -> (-16.225, 73.8076) centre (-16.225, 75.3076) ccw projected
  line L42 (-14.955, 73.8076) -> (-16.225, 73.8076) projected
  arc A46 (-14.955, 72.8076) -> (-14.955, 73.8076) centre (-14.955, 73.3076) ccw projected
  line L43 (-17.725, 72.8076) -> (-14.955, 72.8076) projected
  line L44 (-9.8956, 82.7704) -> (-8.5106, 80.3715) projected
  arc A47 (-9.8956, 82.7704) -> (-12.4937, 81.2704) centre (-11.1947, 82.0204) ccw projected
  line L45 (-11.8587, 80.1705) -> (-12.4937, 81.2704) projected
  arc A48 (-12.1508, 79.4408) -> (-11.8587, 80.1705) centre (-12.2917, 79.9205) ccw projected
  arc A49 (-17.063, 81.9332) -> (-19.5523, 81.7704) centre (-18.2533, 81.0204) ccw projected
  line L46 (-20.1873, 80.6705) -> (-19.5523, 81.7704) projected
  arc A50 (-21.0533, 81.1705) -> (-20.1873, 80.6705) centre (-20.6203, 80.9205) ccw projected
  line L47 (-19.6683, 83.5694) -> (-21.0533, 81.1705) projected
  line L48 (-33.655, 71.8076) -> (-36.425, 71.8076) projected
  arc A51 (-33.655, 71.8076) -> (-33.655, 74.8076) centre (-33.655, 73.3076) ccw projected
  line L49 (-34.925, 74.8076) -> (-33.655, 74.8076) projected
  arc A52 (-35.4109, 75.4254) -> (-34.925, 74.8076) centre (-34.925, 75.3076) ccw projected
  arc A53 (-30.7963, 78.4333) -> (-29.6927, 80.6705) centre (-30.9917, 79.9205) ccw projected
  line L50 (-30.3277, 81.7704) -> (-29.6927, 80.6705) projected
  arc A54 (-29.4617, 82.2704) -> (-30.3277, 81.7704) centre (-29.8947, 82.0204) ccw projected
  line L51 (-28.0767, 79.8715) -> (-29.4617, 82.2704) projected
  line L52 (-40.6194, 81.6705) -> (-39.2344, 84.0694) projected
  arc A55 (-40.6194, 81.6705) -> (-38.0213, 80.1705) centre (-39.3203, 80.9205) ccw projected
  line L53 (-37.3863, 81.2704) -> (-38.0213, 80.1705) projected
  arc A56 (-36.6083, 81.3823) -> (-37.3863, 81.2704) centre (-36.9533, 81.0204) ccw projected
  arc A57 (-36.3107, 75.8819) -> (-34.925, 73.8076) centre (-34.925, 75.3076) ccw projected
  line L54 (-33.655, 73.8076) -> (-34.925, 73.8076) projected
  arc A58 (-33.655, 72.8076) -> (-33.655, 73.8076) centre (-33.655, 73.3076) ccw projected
  line L55 (-36.425, 72.8076) -> (-33.655, 72.8076) projected
  line L56 (-28.5956, 82.7704) -> (-27.2106, 80.3715) projected
  arc A59 (-28.5956, 82.7704) -> (-31.1937, 81.2704) centre (-29.8947, 82.0204) ccw projected
  line L57 (-30.5587, 80.1705) -> (-31.1937, 81.2704) projected
  arc A60 (-30.8508, 79.4408) -> (-30.5587, 80.1705) centre (-30.9917, 79.9205) ccw projected
  arc A61 (-35.763, 81.9332) -> (-38.2523, 81.7704) centre (-36.9533, 81.0204) ccw projected
  line L58 (-38.8873, 80.6705) -> (-38.2523, 81.7704) projected
  arc A62 (-39.7533, 81.1705) -> (-38.8873, 80.6705) centre (-39.3203, 80.9205) ccw projected
  line L59 (-38.3683, 83.5694) -> (-39.7533, 81.1705) projected
  line L60 (-59.3194, 81.6705) -> (-57.9344, 84.0694) projected
  arc A63 (-59.3194, 81.6705) -> (-56.7213, 80.1705) centre (-58.0203, 80.9205) ccw projected
  line L61 (-56.0863, 81.2704) -> (-56.7213, 80.1705) projected
  arc A64 (-55.3083, 81.3823) -> (-56.0863, 81.2704) centre (-55.6533, 81.0204) ccw projected
  arc A65 (-55.0107, 75.8819) -> (-53.625, 73.8076) centre (-53.625, 75.3076) ccw projected
  line L62 (-52.355, 73.8076) -> (-53.625, 73.8076) projected
  arc A66 (-52.355, 72.8076) -> (-52.355, 73.8076) centre (-52.355, 73.3076) ccw projected
  line L63 (-55.125, 72.8076) -> (-52.355, 72.8076) projected
  arc A67 (-54.463, 81.9332) -> (-56.9523, 81.7704) centre (-55.6533, 81.0204) ccw projected
  line L64 (-57.5873, 80.6705) -> (-56.9523, 81.7704) projected
  arc A68 (-58.4533, 81.1705) -> (-57.5873, 80.6705) centre (-58.0203, 80.9205) ccw projected
  line L65 (-57.0683, 83.5694) -> (-58.4533, 81.1705) projected
  line L66 (-47.2956, 82.7704) -> (-45.9106, 80.3715) projected
  arc A69 (-47.2956, 82.7704) -> (-49.8937, 81.2704) centre (-48.5947, 82.0204) ccw projected
  line L67 (-49.2587, 80.1705) -> (-49.8937, 81.2704) projected
  arc A70 (-49.5508, 79.4408) -> (-49.2587, 80.1705) centre (-49.6917, 79.9205) ccw projected
  arc A71 (-49.4963, 78.4333) -> (-48.3927, 80.6705) centre (-49.6917, 79.9205) ccw projected
  line L68 (-49.0277, 81.7704) -> (-48.3927, 80.6705) projected
  arc A72 (-48.1617, 82.2704) -> (-49.0277, 81.7704) centre (-48.5947, 82.0204) ccw projected
  line L69 (-46.7767, 79.8715) -> (-48.1617, 82.2704) projected
  line L70 (-52.355, 71.8076) -> (-55.125, 71.8076) projected
  arc A73 (-52.355, 71.8076) -> (-52.355, 74.8076) centre (-52.355, 73.3076) ccw projected
  line L71 (-53.625, 74.8076) -> (-52.355, 74.8076) projected
  arc A74 (-54.1109, 75.4254) -> (-53.625, 74.8076) centre (-53.625, 75.3076) ccw projected
  line L72 (-3, 66.587) -> (-65.58, 66.587) projected
  line L73 (-3, 104.95) -> (-3, 66.587) projected
  line L74 (-65.58, 104.95) -> (-3, 104.95) projected
  line L75 (-65.58, 66.587) -> (-65.58, 104.95) projected
  arc A75 (-12.1508, 95.6008) -> (-17.063, 98.0932) centre (-15.59, 94.9095) ccw projected
  arc A76 (-22.7854, 98.3305) -> (-22.6297, 95.5931) centre (-20.6203, 97.0805) ccw projected
  line L76 (-21.4004, 100.7294) -> (-22.7854, 98.3305) projected
  line L77 (-20.5344, 100.2294) -> (-21.4004, 100.7294) projected
  arc A77 (-9.0296, 99.4304) -> (-11.4782, 100.6643) centre (-11.1947, 98.1804) ccw projected
  line L78 (-7.6446, 97.0315) -> (-9.0296, 99.4304) projected
  line L79 (-8.5106, 96.5315) -> (-7.6446, 97.0315) projected
  arc A78 (-14.955, 86.9676) -> (-12.6621, 88.4712) centre (-14.955, 89.4676) ccw projected
  line L80 (-17.725, 86.9676) -> (-14.955, 86.9676) projected
  line L81 (-17.725, 87.9676) -> (-17.725, 86.9676) projected
  arc A79 (-30.8508, 95.6008) -> (-35.763, 98.0932) centre (-34.29, 94.9095) ccw projected
  arc A80 (-41.4854, 98.3305) -> (-41.3297, 95.5931) centre (-39.3203, 97.0805) ccw projected
  line L82 (-40.1004, 100.7294) -> (-41.4854, 98.3305) projected
  line L83 (-39.2344, 100.2294) -> (-40.1004, 100.7294) projected
  arc A81 (-27.7296, 99.4304) -> (-30.1782, 100.6643) centre (-29.8947, 98.1804) ccw projected
  line L84 (-26.3446, 97.0315) -> (-27.7296, 99.4304) projected
  line L85 (-27.2106, 96.5315) -> (-26.3446, 97.0315) projected
  arc A82 (-33.655, 86.9676) -> (-31.3621, 88.4712) centre (-33.655, 89.4676) ccw projected
  line L86 (-36.425, 86.9676) -> (-33.655, 86.9676) projected
  line L87 (-36.425, 87.9676) -> (-36.425, 86.9676) projected
  arc A83 (-49.5508, 95.6008) -> (-54.463, 98.0932) centre (-52.99, 94.9095) ccw projected
  arc A84 (-60.1854, 98.3305) -> (-60.0297, 95.5931) centre (-58.0203, 97.0805) ccw projected
  line L88 (-58.8004, 100.7294) -> (-60.1854, 98.3305) projected
  line L89 (-57.9344, 100.2294) -> (-58.8004, 100.7294) projected
  arc A85 (-46.4296, 99.4304) -> (-48.8782, 100.6643) centre (-48.5947, 98.1804) ccw projected
  line L90 (-45.0446, 97.0315) -> (-46.4296, 99.4304) projected
  line L91 (-45.9106, 96.5315) -> (-45.0446, 97.0315) projected
  arc A86 (-52.355, 86.9676) -> (-50.0621, 88.4712) centre (-52.355, 89.4676) ccw projected
  line L92 (-55.125, 86.9676) -> (-52.355, 86.9676) projected
  line L93 (-55.125, 87.9676) -> (-55.125, 86.9676) projected
  arc A87 (-12.1508, 79.4408) -> (-17.063, 81.9332) centre (-15.59, 78.7495) ccw projected
  arc A88 (-22.7854, 82.1705) -> (-22.6297, 79.4331) centre (-20.6203, 80.9205) ccw projected
  line L94 (-21.4004, 84.5694) -> (-22.7854, 82.1705) projected
  line L95 (-20.5344, 84.0694) -> (-21.4004, 84.5694) projected
  arc A89 (-9.0296, 83.2704) -> (-11.4782, 84.5043) centre (-11.1947, 82.0204) ccw projected
  line L96 (-7.6446, 80.8715) -> (-9.0296, 83.2704) projected
  line L97 (-8.5106, 80.3715) -> (-7.6446, 80.8715) projected
  arc A90 (-14.955, 70.8076) -> (-12.6621, 72.3112) centre (-14.955, 73.3076) ccw projected
  line L98 (-17.725, 70.8076) -> (-14.955, 70.8076) projected
  line L99 (-17.725, 71.8076) -> (-17.725, 70.8076) projected
  arc A91 (-30.8508, 79.4408) -> (-35.763, 81.9332) centre (-34.29, 78.7495) ccw projected
  arc A92 (-41.4854, 82.1705) -> (-41.3297, 79.4331) centre (-39.3203, 80.9205) ccw projected
  line L100 (-40.1004, 84.5694) -> (-41.4854, 82.1705) projected
  line L101 (-39.2344, 84.0694) -> (-40.1004, 84.5694) projected
  arc A93 (-27.7296, 83.2704) -> (-30.1782, 84.5043) centre (-29.8947, 82.0204) ccw projected
  line L102 (-26.3446, 80.8715) -> (-27.7296, 83.2704) projected
  line L103 (-27.2106, 80.3715) -> (-26.3446, 80.8715) projected
  arc A94 (-33.655, 70.8076) -> (-31.3621, 72.3112) centre (-33.655, 73.3076) ccw projected
  line L104 (-36.425, 70.8076) -> (-33.655, 70.8076) projected
  line L105 (-36.425, 71.8076) -> (-36.425, 70.8076) projected
  arc A95 (-46.4296, 83.2704) -> (-48.8782, 84.5043) centre (-48.5947, 82.0204) ccw projected
  line L106 (-45.0446, 80.8715) -> (-46.4296, 83.2704) projected
  line L107 (-45.9106, 80.3715) -> (-45.0446, 80.8715) projected
  arc A96 (-52.355, 70.8076) -> (-50.0621, 72.3112) centre (-52.355, 73.3076) ccw projected
  line L108 (-55.125, 70.8076) -> (-52.355, 70.8076) projected
  line L109 (-55.125, 71.8076) -> (-55.125, 70.8076) projected
  arc A97 (-60.1854, 82.1705) -> (-60.0297, 79.4331) centre (-58.0203, 80.9205) ccw projected
  line L110 (-58.8004, 84.5694) -> (-60.1854, 82.1705) projected
  line L111 (-57.9344, 84.0694) -> (-58.8004, 84.5694) projected
  arc A98 (-17.9083, 97.5423) -> (-17.6107, 92.0419) centre (-15.59, 94.9095) ccw projected
  arc A99 (-36.6083, 97.5423) -> (-36.3107, 92.0419) centre (-34.29, 94.9095) ccw projected
  arc A100 (-55.3083, 97.5423) -> (-55.0107, 92.0419) centre (-52.99, 94.9095) ccw projected
  arc A101 (-17.9083, 81.3823) -> (-17.6107, 75.8819) centre (-15.59, 78.7495) ccw projected
  arc A102 (-36.6083, 81.3823) -> (-36.3107, 75.8819) centre (-34.29, 78.7495) ccw projected
  line L112 (-12.6621, 88.4712) -> (-9.3767, 96.0315) projected
  arc A103 (-16.7109, 91.5854) -> (-12.0963, 94.5933) centre (-15.59, 94.9095) ccw projected
  line L113 (-31.3621, 88.4712) -> (-28.0767, 96.0315) projected
  arc A104 (-35.4109, 91.5854) -> (-30.7963, 94.5933) centre (-34.29, 94.9095) ccw projected
  line L114 (-50.0621, 88.4712) -> (-46.7767, 96.0315) projected
  arc A105 (-54.1109, 91.5854) -> (-49.4963, 94.5933) centre (-52.99, 94.9095) ccw projected
  line L115 (-12.6621, 72.3112) -> (-9.3767, 79.8715) projected
  arc A106 (-16.7109, 75.4254) -> (-12.0963, 78.4333) centre (-15.59, 78.7495) ccw projected
  line L116 (-31.3621, 72.3112) -> (-28.0767, 79.8715) projected
  arc A107 (-35.4109, 75.4254) -> (-30.7963, 78.4333) centre (-34.29, 78.7495) ccw projected
  line L117 (-48.8782, 84.5043) -> (-57.0683, 83.5694) projected
  arc A108 (-49.5508, 79.4408) -> (-54.463, 81.9332) centre (-52.99, 78.7495) ccw projected
  line L118 (-60.0297, 79.4331) -> (-55.125, 72.8076) projected
  arc A109 (-55.3083, 81.3823) -> (-55.0107, 75.8819) centre (-52.99, 78.7495) ccw projected
  line L119 (-50.0621, 72.3112) -> (-46.7767, 79.8715) projected
  arc A110 (-54.1109, 75.4254) -> (-49.4963, 78.4333) centre (-52.99, 78.7495) ccw projected
  line L120 (-22.6297, 95.5931) -> (-17.725, 88.9676) projected
  line L121 (-41.3297, 95.5931) -> (-36.425, 88.9676) projected
  line L122 (-60.0297, 95.5931) -> (-55.125, 88.9676) projected
  line L123 (-22.6297, 79.4331) -> (-17.725, 72.8076) projected
  line L124 (-41.3297, 79.4331) -> (-36.425, 72.8076) projected
  line L125 (-11.4782, 100.6643) -> (-19.6683, 99.7294) projected
  line L126 (-30.1782, 100.6643) -> (-38.3683, 99.7294) projected
  line L127 (-48.8782, 100.6643) -> (-57.0683, 99.7294) projected
  line L128 (-11.4782, 84.5043) -> (-19.6683, 83.5694) projected
  line L129 (-30.1782, 84.5043) -> (-38.3683, 83.5694) projected
  line L130 (-28.0767, 96.0315) -> (-27.2106, 96.5315)
  line L131 (-21.9194, 97.8305) -> (-20.5344, 100.2294) projected
  line L132 (-20.5344, 100.2294) -> (-19.6683, 99.7294)
  line L133 (-12.6621, 88.4712) -> (-9.3767, 96.0315) projected
  line L134 (-9.8956, 98.9304) -> (-8.5106, 96.5315) projected
  line L135 (-9.3767, 96.0315) -> (-8.5106, 96.5315)
  line L136 (-17.725, 87.9676) -> (-17.725, 88.9676)
  line L137 (-36.425, 87.9676) -> (-36.425, 86.9676) projected
  line L138 (-41.3297, 95.5931) -> (-36.425, 88.9676) projected
  line L139 (-36.425, 87.9676) -> (-36.425, 88.9676)
  line L140 (-30.1782, 100.6643) -> (-38.3683, 99.7294) projected
  line L141 (-39.2344, 100.2294) -> (-38.3683, 99.7294)
  line L142 (-50.0621, 88.4712) -> (-46.7767, 96.0315) projected
  line L143 (-46.7767, 96.0315) -> (-45.9106, 96.5315)
  line L144 (-57.0683, 99.7294) -> (-57.9344, 100.2294)
  line L145 (-60.0297, 95.5931) -> (-55.125, 88.9676) projected
  line L146 (-55.125, 88.9676) -> (-55.125, 87.9676)
  line L147 (-57.9344, 84.0694) -> (-57.0683, 83.5694)
  line L148 (-57.0683, 83.5694) -> (-58.4533, 81.1705) projected
  line L149 (-46.7767, 79.8715) -> (-45.9106, 80.3715)
  line L150 (-55.125, 71.8076) -> (-55.125, 72.8076)
  line L151 (-39.2344, 84.0694) -> (-40.1004, 84.5694) projected
  line L152 (-39.2344, 84.0694) -> (-38.3683, 83.5694)
  line L153 (-28.0767, 79.8715) -> (-27.2106, 80.3715)
  line L154 (-36.425, 72.8076) -> (-36.425, 71.8076)
  line L155 (-17.725, 72.8076) -> (-17.725, 71.8076)
  line L156 (-9.3767, 79.8715) -> (-10.7617, 82.2704) projected
  line L157 (-9.3767, 79.8715) -> (-8.5106, 80.3715)
  line L158 (-21.9194, 81.6705) -> (-20.5344, 84.0694) projected
  line L159 (-20.5344, 84.0694) -> (-19.6683, 83.5694)
  point P0 (0, 0)
  constraints: 36 end point, 5 perpendicular, 5 vertical, 2 collinear
extrude "Extrusion10" add sketch "Sketch8" along normal blind 4.9
fillet "Fillet1" radius 5 4 edges at (68.58, 107.95, 5) (0, 107.95, 5) (0, 0, 5) (68.58, 0, 5)
chamfer "Chamfer1" distance 2 angle 45 8 edges at (34.29, 0, 10) (67.1155, 1.4645, 10) (68.58, 53.975, 10) (67.1155, 106.4855, 10) (34.29, 107.95, 10) (1.4645, 106.4855, 10) (0, 53.975, 10) (1.4645, 1.4645, 10)
sketch "Sketch9" plane through (34.29, 35.56, 4) normal (0, 0, 1) x (1, 0, 0)
  line L0 (0, 25.4139) -> (22.0091, -12.707) construction
  line L1 (22.0091, -12.707) -> (-22.0091, -12.707) construction
  line L2 (-22.0091, -12.707) -> (0, 25.4139) construction
  circle A0 centre (0, 25.4139) radius 2
  circle A1 centre (22.0091, -12.707) radius 2
  circle A2 centre (-22.0091, -12.707) radius 2
  circle A3 centre (0, 0) radius 21.3606 projected
  point P0 (-34.29, -35.56)
  dimension "d94" = 44.0182
  dimension "d95" = 4
  constraints: 6 end point, 4 coincident, 3 centre point, 2 equal radius, 1 horizontal, 7 other
  measures "d94" distance of L0.start L0.end
  measures "d95" diameter of A2
extrude "Extrusion11" cut sketch "Sketch9" against normal through all contours A0 | A1 | A2